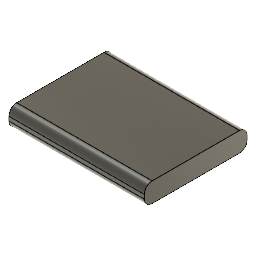
1317 150mAh Lipo Battery (Autodesk Fusion 360 design; units mm, degrees)
Autodesk Fusion 360 part; units mm, degrees
sketch "Sketch1" plane through (0, 0, 0) normal (0, 0, 1) x (1, 0, 0)
  line L0 (0, 0) -> (26.02, 0)
  line L1 (26.02, 0) -> (26.02, 19.75)
  line L2 (26.02, 19.75) -> (0, 19.75)
  line L3 (0, 19.75) -> (0, 0)
  dimension "d1" = 26.02
  dimension "d2" = 19.75
  measures "d2" distance of L0.start
extrude "Extrude1" add sketch "Sketch1" along normal blind 3.8
fillet "Fillet1" radius 1.5 4 edges at (13.01, 0, 3.8) (13.01, 0, 0) (13.01, 19.75, 3.8) (13.01, 19.75, 0)
